Autodesk Fusion 360 part; units mm, degrees
(part 11 of 25)
  arc A1929 (12.5422, 52.0786) -> (12.3177, 51.8541) centre (12.4299, 51.9664) ccw
  arc A1930 (17.6222, 52.0786) -> (17.3977, 51.8541) centre (17.5099, 51.9664) ccw
  line L597 (17.9596, 51.5167) -> (17.51, 51.9663)
  arc A1931 (6.3546, 45.2309) -> (6.0612, 45.3524) centre (6.2079, 45.2917) ccw
  line L598 (10.4521, 47.0845) -> (10.4521, 46.1251)
  arc A1932 (9.1447, 46.0826) -> (9.0232, 45.7892) centre (9.084, 45.9359) ccw
  arc A1933 (18.1777, 51.5103) -> (17.9532, 51.7348) centre (18.0654, 51.6226) ccw
  arc A1934 (5.8229, 44.1544) -> (6.1405, 44.1544) centre (5.9817, 44.1544) ccw
  arc A1935 (9.084, 45.7771) -> (9.084, 46.0946) centre (9.084, 45.9359) ccw
  arc A1936 (17.8473, 51.629) -> (18.0719, 51.4044) centre (17.9596, 51.5167) ccw
  arc A1937 (9.7212, 45.6186) -> (9.9457, 45.3941) centre (9.8334, 45.5063) ccw
  arc A1938 (17.8473, 51.4044) -> (18.0719, 51.629) centre (17.9596, 51.5167) ccw
  arc A1939 (9.0232, 40.5708) -> (9.1447, 40.2774) centre (9.084, 40.4241) ccw
  arc A1940 (6.1405, 42.2056) -> (5.8229, 42.2056) centre (5.9817, 42.2056) ccw
  arc A1941 (9.7212, 45.3941) -> (9.9457, 45.6186) centre (9.8334, 45.5063) ccw
  line L599 (10.4521, 46.1251) -> (9.8334, 45.5064)
  line L600 (13.6189, 52.2351) -> (12.97, 51.9663)
  line L601 (7.172, 40.4241) -> (9.084, 40.4241)
  line L602 (6.6259, 45.7097) -> (6.2079, 45.2917)
  line L603 (5.9817, 44.7456) -> (5.9817, 44.1544)
  arc A1942 (6.5901, 43.0333) -> (6.7116, 43.3267) centre (6.6508, 43.18) ccw
  line L604 (6.6259, 43.1903) -> (6.6508, 43.18)
  arc A1943 (6.0957, 45.4039) -> (6.3202, 45.1794) centre (6.208, 45.2917) ccw
  line L605 (9.6301, 45.7097) -> (9.084, 45.9359)
  arc A1944 (10.3693, 52.113) -> (10.4908, 51.8197) centre (10.4301, 51.9664) ccw
  line L606 (15.51, 51.9663) -> (15.24, 51.6963)
  arc A1945 (6.5652, 45.8563) -> (6.6867, 45.563) centre (6.626, 45.7097) ccw
  line L607 (7.172, 45.9359) -> (6.6259, 45.7097)
  arc A1946 (6.3202, 41.1806) -> (6.0957, 40.956) centre (6.208, 41.0683) ccw
  line L608 (9.084, 45.9359) -> (7.172, 45.9359)
  arc A1947 (6.7116, 43.0333) -> (6.5901, 43.3267) centre (6.6508, 43.18) ccw
  arc A1948 (12.5877, 51.8086) -> (12.8123, 51.5841) centre (12.7, 51.6963) ccw
  line L609 (16.1589, 52.2351) -> (15.51, 51.9663)
  arc A1949 (6.5136, 43.0781) -> (6.7382, 43.3026) centre (6.6259, 43.1904) ccw
  line L610 (9.8334, 45.5064) -> (9.6301, 45.7097)
  line L611 (6.2079, 45.2917) -> (5.9817, 44.7456)
  arc A1950 (9.5693, 45.563) -> (9.6908, 45.8563) centre (9.6301, 45.7097) ccw
  arc A1951 (5.835, 44.8063) -> (6.1284, 44.6848) centre (5.9817, 44.7456) ccw
  arc A1952 (6.1284, 44.2152) -> (5.835, 44.0937) centre (5.9817, 44.1544) ccw
  arc A1953 (14.3819, 52.3818) -> (14.2604, 52.0884) centre (14.3211, 52.2351) ccw
  arc A1954 (15.0822, 52.0786) -> (14.8577, 51.8541) centre (14.9699, 51.9664) ccw
  arc A1955 (15.1277, 51.8086) -> (15.3523, 51.5841) centre (15.24, 51.6963) ccw
  line L612 (11.0789, 52.2351) -> (10.43, 51.9663)
  arc A1956 (7.2328, 45.7892) -> (7.1113, 46.0826) centre (7.1721, 45.9359) ccw
  arc A1957 (6.0612, 43.5476) -> (6.3546, 43.6691) centre (6.2079, 43.6084) ccw
  line L613 (6.6259, 43.1697) -> (6.2079, 42.7517)
  line L614 (6.6508, 43.18) -> (6.6259, 43.1697)
  arc A1958 (9.6908, 40.5036) -> (9.5693, 40.797) centre (9.6301, 40.6503) ccw
  arc A1959 (11.0789, 52.3938) -> (11.0789, 52.0763) centre (11.0789, 52.2351) ccw
  line L615 (9.084, 40.4241) -> (9.6301, 40.6503)
  arc A1960 (6.3202, 43.7206) -> (6.0957, 43.496) centre (6.2079, 43.6083) ccw
  line L616 (5.9817, 44.1544) -> (6.2079, 43.6083)
  arc A1961 (9.084, 40.2654) -> (9.084, 40.5829) centre (9.084, 40.4241) ccw
  line L617 (5.9817, 42.2056) -> (5.9817, 41.6144)
  arc A1962 (6.6867, 40.797) -> (6.5652, 40.5036) centre (6.626, 40.6503) ccw
  line L618 (14.3211, 52.2351) -> (13.6189, 52.2351)
  arc A1963 (7.172, 40.5829) -> (7.172, 40.2654) centre (7.172, 40.4241) ccw
  arc A1964 (10.4908, 47.2403) -> (10.3693, 46.947) centre (10.43, 47.0936) ccw
  line L619 (12.97, 51.9663) -> (12.7, 51.6963)
  arc A1965 (12.9093, 52.113) -> (13.0308, 51.8197) centre (12.9701, 51.9664) ccw
  line L620 (12.43, 51.9663) -> (11.7811, 52.2351)
  arc A1966 (14.9092, 51.8197) -> (15.0307, 52.113) centre (14.97, 51.9663) ccw
  arc A1967 (12.5877, 51.5841) -> (12.8123, 51.8086) centre (12.7, 51.6964) ccw
  arc A1968 (10.5644, 46.0128) -> (10.3398, 46.2373) centre (10.4521, 46.1251) ccw
  arc A1969 (7.172, 46.0946) -> (7.172, 45.7771) centre (7.172, 45.9359) ccw
  line L621 (11.7811, 52.2351) -> (11.0789, 52.2351)
  arc A1970 (14.2402, 42.552) -> (14.3617, 42.2586) centre (14.3009, 42.4053) ccw
  line L622 (6.6259, 35.5497) -> (6.3441, 35.2679)
  arc A1971 (15.746, 44.0556) -> (15.5214, 43.8311) centre (15.6337, 43.9434) ccw
  line L623 (10.7139, 41.081) -> (12.6596, 43.0266)
  arc A1972 (9.9358, 35.0194) -> (10.1603, 35.2439) centre (10.0481, 35.1317) ccw
  arc A1973 (7.1113, 40.2774) -> (7.2328, 40.5708) centre (7.1721, 40.4241) ccw
  arc A1974 (6.5652, 43.3164) -> (6.6866, 43.023) centre (6.6259, 43.1697) ccw
  arc A1975 (6.7382, 45.5974) -> (6.5136, 45.8219) centre (6.6259, 45.7097) ccw
  arc A1976 (9.7423, 45.8219) -> (9.5178, 45.5974) centre (9.63, 45.7097) ccw
  arc A1977 (10.6108, 47.0845) -> (10.2934, 47.0845) centre (10.4521, 47.0845) ccw
  arc A1978 (9.1447, 35.9226) -> (9.0232, 35.6292) centre (9.084, 35.7759) ccw
  arc A1979 (14.8002, 42.7708) -> (15.0247, 42.5463) centre (14.9124, 42.6586) ccw
  arc A1980 (5.835, 42.2663) -> (6.1284, 42.1448) centre (5.9817, 42.2056) ccw
  line L624 (13.4861, 31.4579) -> (10.2148, 34.7291)
  arc A1981 (6.6867, 43.337) -> (6.5651, 43.0437) centre (6.6259, 43.1904) ccw
  line L625 (13.6391, 42.4053) -> (14.3009, 42.4053)
  arc A1982 (9.5693, 35.403) -> (9.6908, 35.6963) centre (9.6301, 35.5496) ccw
  arc A1983 (15.8984, 32.2968) -> (15.6738, 32.5213) centre (15.7861, 32.409) ccw
  line L626 (6.2079, 43.6083) -> (6.6259, 43.1903)
  arc A1984 (14.8349, 31.2991) -> (14.8349, 31.6166) centre (14.8349, 31.4579) ccw
  arc A1985 (6.3546, 42.6909) -> (6.0612, 42.8124) centre (6.2079, 42.7516) ccw
  arc A1986 (9.9119, 41.0909) -> (9.9119, 40.7734) centre (9.9119, 40.9322) ccw
  arc A1987 (6.1405, 44.7456) -> (5.8229, 44.7456) centre (5.9817, 44.7456) ccw
  arc A1988 (6.1284, 41.6752) -> (5.835, 41.5537) centre (5.9817, 41.6144) ccw
  line L627 (9.6301, 35.5497) -> (9.084, 35.7759)
  line L628 (13.0276, 42.6586) -> (13.6391, 42.4053)
  line L629 (5.9817, 41.6144) -> (6.2079, 41.0683)
  line L630 (15.6337, 43.7381) -> (15.6337, 43.9433)
  line L631 (15.7861, 32.4091) -> (14.8349, 31.4579)
  line L632 (9.6301, 40.6503) -> (9.9119, 40.9321)
  line L633 (10.2148, 34.7291) -> (10.0481, 35.1317)
  arc A1989 (6.0957, 42.8639) -> (6.3202, 42.6394) centre (6.208, 42.7517) ccw
  arc A1990 (10.1947, 35.1924) -> (9.9014, 35.0709) centre (10.0481, 35.1317) ccw
  line L634 (9.084, 35.7759) -> (7.172, 35.7759)
  line L635 (6.6259, 40.6503) -> (7.172, 40.4241)
  arc A1991 (7.172, 35.9346) -> (7.172, 35.6171) centre (7.172, 35.7759) ccw
  line L636 (15.3804, 43.1266) -> (15.6337, 43.7381)
  arc A1992 (6.5652, 35.6963) -> (6.6867, 35.403) centre (6.626, 35.5496) ccw
  arc A1993 (6.0612, 41.0076) -> (6.3546, 41.1291) centre (6.2079, 41.0684) ccw
  arc A1994 (10.2934, 46.1251) -> (10.6108, 46.1251) centre (10.4521, 46.1251) ccw
  arc A1995 (10.6017, 41.1932) -> (10.8262, 40.9687) centre (10.714, 41.081) ccw
  arc A1996 (13.6391, 42.5641) -> (13.6391, 42.2466) centre (13.6391, 42.4054) ccw
  arc A1997 (6.5136, 40.5381) -> (6.7382, 40.7626) centre (6.6259, 40.6504) ccw
  line L637 (6.2079, 41.0683) -> (6.6259, 40.6503)
  arc A1998 (6.7382, 43.0574) -> (6.5136, 43.2819) centre (6.6259, 43.1696) ccw
  arc A1999 (10.3545, 40.7734) -> (10.3545, 41.0909) centre (10.3545, 40.9322) ccw
  arc A2000 (14.7227, 31.5702) -> (14.9472, 31.3456) centre (14.8349, 31.4579) ccw
  arc A2001 (13.4861, 31.6166) -> (13.4861, 31.2991) centre (13.4861, 31.4579) ccw
  arc A2002 (12.7718, 42.9144) -> (12.5473, 43.1389) centre (12.6596, 43.0267) ccw
  arc A2003 (15.4927, 43.0143) -> (15.2682, 43.2388) centre (15.3804, 43.1265) ccw
  arc A2004 (5.8229, 41.6144) -> (6.1405, 41.6144) centre (5.9817, 41.6144) ccw
  line L638 (7.172, 35.7759) -> (6.6259, 35.5497)
  arc A2005 (14.9732, 42.5119) -> (14.8517, 42.8052) centre (14.9125, 42.6586) ccw
  line L639 (6.2079, 42.7517) -> (5.9817, 42.2056)
  arc A2006 (9.084, 35.6171) -> (9.084, 35.9346) centre (9.084, 35.7759) ccw
  arc A2007 (7.2328, 35.6292) -> (7.1113, 35.9226) centre (7.172, 35.7759) ccw
  arc A2008 (13.0883, 42.8052) -> (12.9668, 42.5119) centre (13.0276, 42.6586) ccw
  arc A2009 (15.6738, 43.6787) -> (15.8984, 43.9032) centre (15.7861, 43.7909) ccw
  arc A2010 (15.7924, 43.9433) -> (15.4749, 43.9433) centre (15.6337, 43.9433) ccw
  arc A2011 (10.2938, 41.0788) -> (10.4153, 40.7854) centre (10.3546, 40.9321) ccw
  line L640 (21.8221, 44.4397) -> (21.276, 44.6659)
  line L641 (9.9119, 40.9321) -> (10.3545, 40.9321)
  arc A2012 (9.7423, 35.6619) -> (9.5178, 35.4374) centre (9.6301, 35.5496) ccw
  arc A2013 (22.3867, 44.0824) -> (22.0934, 43.9609) centre (22.2401, 44.0217) ccw
  line L642 (10.0481, 35.1317) -> (9.6301, 35.5497)
  line L643 (15.6337, 43.9433) -> (15.7861, 43.7909)
  arc A2014 (10.0682, 34.6684) -> (10.3615, 34.7899) centre (10.2149, 34.7292) ccw
  line L644 (14.8349, 31.4579) -> (13.4861, 31.4579)
  line L645 (10.3545, 40.9321) -> (10.7139, 41.081)
  arc A2015 (15.4749, 43.7381) -> (15.7924, 43.7381) centre (15.6337, 43.7381) ccw
  line L646 (14.9124, 42.6586) -> (15.3804, 43.1266)
  arc A2016 (14.3009, 42.2466) -> (14.3009, 42.5641) centre (14.3009, 42.4054) ccw
  arc A2017 (21.7613, 44.293) -> (21.8828, 44.5863) centre (21.8221, 44.4397) ccw
  arc A2018 (28.3146, 42.5255) -> (27.9971, 42.5255) centre (28.1559, 42.5255) ccw
  arc A2019 (25.3429, 42.5255) -> (25.0253, 42.5255) centre (25.1841, 42.5255) ccw
  line L647 (12.6596, 43.0266) -> (13.0276, 42.6586)
  arc A2020 (21.7364, 42.0567) -> (21.8579, 41.7633) centre (21.7972, 41.91) ccw
  line L648 (21.276, 44.6659) -> (19.364, 44.6659)
  arc A2021 (25.0718, 42.6377) -> (25.2964, 42.4132) centre (25.1841, 42.5255) ccw
  arc A2022 (10.3271, 34.8414) -> (10.1026, 34.6169) centre (10.2149, 34.7292) ccw
  line L649 (22.1039, 41.6179) -> (21.8221, 41.8997)
  arc A2023 (22.3196, 43.4148) -> (22.613, 43.5363) centre (22.4663, 43.4755) ccw
  line L650 (14.3009, 42.4053) -> (14.9124, 42.6586)
  arc A2024 (21.276, 44.5071) -> (21.276, 44.8246) centre (21.276, 44.6658) ccw
  arc A2025 (15.6274, 32.4091) -> (15.9449, 32.4091) centre (15.7862, 32.4091) ccw
  line L651 (15.7861, 43.7909) -> (15.7861, 32.4091)
  arc A2026 (13.3738, 31.3456) -> (13.5983, 31.5702) centre (13.4861, 31.4579) ccw
  arc A2027 (9.5178, 40.7626) -> (9.7423, 40.5381) centre (9.63, 40.6504) ccw
  arc A2028 (25.0253, 41.8071) -> (25.3429, 41.8071) centre (25.1841, 41.8071) ccw
  arc A2029 (21.7098, 42.0326) -> (21.9343, 41.8081) centre (21.8221, 41.9204) ccw
  line L652 (4.8319, 35.2679) -> (4.5501, 35.5497)
  arc A2030 (12.7718, 43.1389) -> (12.5473, 42.9144) centre (12.6595, 43.0267) ccw
  arc A2031 (21.9343, 42.0119) -> (21.7098, 41.7874) centre (21.8221, 41.8997) ccw
  arc A2032 (10.7747, 40.9343) -> (10.6532, 41.2276) centre (10.7139, 41.081) ccw
  line L653 (22.4663, 42.8844) -> (22.4663, 43.4756)
  arc A2033 (10.0241, 40.8198) -> (9.7996, 41.0444) centre (9.9119, 40.9321) ccw
  line L654 (25.1841, 41.8071) -> (24.9949, 41.6179)
  arc A2034 (15.9449, 43.7909) -> (15.6274, 43.7909) centre (15.7862, 43.7909) ccw
  arc A2035 (6.7382, 35.4374) -> (6.5136, 35.6619) centre (6.6259, 35.5496) ccw
  arc A2036 (4.4893, 35.403) -> (4.6108, 35.6963) centre (4.5501, 35.5496) ccw
  arc A2037 (21.9916, 41.5056) -> (22.2161, 41.7301) centre (22.1038, 41.6179) ccw
  arc A2038 (21.9343, 44.5519) -> (21.7098, 44.3274) centre (21.822, 44.4397) ccw
  line L655 (22.2401, 44.0217) -> (21.8221, 44.4397)
  arc A2039 (19.364, 44.8246) -> (19.364, 44.5071) centre (19.364, 44.6658) ccw
  arc A2040 (13.5783, 42.2586) -> (13.6998, 42.552) centre (13.639, 42.4053) ccw
  arc A2041 (12.9153, 42.5463) -> (13.1398, 42.7708) centre (13.0275, 42.6586) ccw
  arc A2042 (15.7804, 43.6773) -> (15.487, 43.7988) centre (15.6337, 43.7381) ccw
  arc A2043 (4.6623, 35.6619) -> (4.4378, 35.4374) centre (4.55, 35.5497) ccw
  arc A2044 (6.2319, 35.3802) -> (6.4564, 35.1556) centre (6.3441, 35.2679) ccw
  line L656 (4.5501, 35.5497) -> (4.004, 35.7759)
  arc A2045 (15.2337, 43.1873) -> (15.5271, 43.0658) centre (15.3804, 43.1266) ccw
  arc A2046 (21.3367, 44.8126) -> (21.2152, 44.5192) centre (21.2759, 44.6659) ccw
  arc A2047 (4.7196, 35.1556) -> (4.9441, 35.3802) centre (4.8319, 35.2679) ccw
  arc A2048 (22.613, 42.8237) -> (22.3196, 42.9452) centre (22.4663, 42.8845) ccw
  arc A2049 (18.9302, 44.3274) -> (18.7056, 44.5519) centre (18.8179, 44.4396) ccw
  arc A2050 (18.7572, 44.5863) -> (18.8787, 44.293) centre (18.8179, 44.4397) ccw
  line L657 (28.1559, 42.5255) -> (27.2855, 43.3959)
  line L658 (25.1841, 42.5255) -> (25.1841, 41.8071)
  arc A2051 (21.8828, 41.7736) -> (21.7614, 42.067) centre (21.8221, 41.9203) ccw
  line L659 (27.2855, 43.3959) -> (26.0545, 43.3959)
  line L660 (6.3441, 35.2679) -> (4.8319, 35.2679)
  line L661 (21.8221, 41.8997) -> (21.7972, 41.91)
  arc A2052 (21.7613, 41.753) -> (21.8828, 42.0463) centre (21.8221, 41.8997) ccw
  arc A2053 (22.1039, 41.7766) -> (22.1039, 41.4591) centre (22.1039, 41.6179) ccw
  arc A2054 (22.3523, 42.226) -> (22.1278, 42.4506) centre (22.24, 42.3383) ccw
  line L662 (24.9949, 41.6179) -> (22.1039, 41.6179)
  arc A2055 (22.0934, 42.3991) -> (22.3867, 42.2776) centre (22.2401, 42.3383) ccw
  arc A2056 (28.0436, 42.4132) -> (28.2682, 42.6377) centre (28.1559, 42.5255) ccw
  arc A2057 (22.3075, 42.8844) -> (22.625, 42.8844) centre (22.4663, 42.8844) ccw
  arc A2058 (4.0647, 35.9226) -> (3.9432, 35.6292) centre (4.004, 35.7759) ccw
  arc A2059 (6.3441, 35.1091) -> (6.3441, 35.4266) centre (6.3441, 35.2678) ccw
  arc A2060 (18.5466, 41.4209) -> (18.2532, 41.5424) centre (18.3999, 41.4817) ccw
  arc A2061 (18.3325, 43.4756) -> (18.0149, 43.4756) centre (18.1737, 43.4756) ccw
  arc A2062 (27.9971, 41.2945) -> (28.3146, 41.2945) centre (28.1559, 41.2945) ccw
  arc A2063 (24.9949, 41.4591) -> (24.9949, 41.7766) centre (24.9949, 41.6179) ccw
  arc A2064 (4.8319, 35.4266) -> (4.8319, 35.1091) centre (4.8319, 35.2678) ccw
  arc A2065 (18.3765, 38.645) -> (18.6594, 38.5008) centre (18.5179, 38.5729) ccw
  line L663 (18.8179, 41.8997) -> (18.3999, 41.4817)
  arc A2066 (18.7474, 38.6736) -> (18.4645, 38.8177) centre (18.606, 38.7457) ccw
  line L664 (18.458, 38.3885) -> (18.4277, 38.197)
  line L665 (21.7972, 41.91) -> (21.8221, 41.9203)
  arc A2067 (22.1278, 43.9094) -> (22.3523, 44.1339) centre (22.2401, 44.0217) ccw
  arc A2068 (27.2855, 43.2371) -> (27.2855, 43.5546) centre (27.2855, 43.3959) ccw
  arc A2069 (18.5865, 38.197) -> (18.269, 38.197) centre (18.4277, 38.197) ccw
  arc A2070 (27.3977, 43.5082) -> (27.1732, 43.2836) centre (27.2855, 43.3959) ccw
  arc A2071 (18.5122, 42.4506) -> (18.2877, 42.226) centre (18.4, 42.3383) ccw
  line L666 (18.4277, 38.197) -> (18.4277, 38.1)
  line L667 (21.8221, 41.9203) -> (22.2401, 42.3383)
  arc A2072 (19.1107, 39.0872) -> (19.2322, 39.3805) centre (19.1715, 39.2339) ccw
  line L668 (26.0545, 43.3959) -> (25.1841, 42.5255)
  arc A2073 (18.3204, 42.9452) -> (18.027, 42.8237) centre (18.1737, 42.8845) ccw
  arc A2074 (24.8827, 41.7302) -> (25.1072, 41.5056) centre (24.9949, 41.6179) ccw
  line L669 (18.8571, 39.0396) -> (18.72, 38.9025)
  arc A2075 (18.8786, 42.067) -> (18.7572, 41.7736) centre (18.8179, 41.9203) ccw
  line L670 (28.1559, 41.2945) -> (28.1559, 42.5255)
  line L671 (19.364, 44.6659) -> (18.8179, 44.4397)
  arc A2076 (26.0545, 43.5546) -> (26.0545, 43.2371) centre (26.0545, 43.3959) ccw
  line L672 (22.2401, 42.3383) -> (22.4663, 42.8844)
  arc A2077 (22.625, 43.4756) -> (22.3075, 43.4756) centre (22.4663, 43.4756) ccw
  arc A2078 (26.1668, 43.2836) -> (25.9423, 43.5082) centre (26.0545, 43.3959) ccw
  arc A2079 (18.2877, 44.1339) -> (18.5122, 43.9094) centre (18.4, 44.0217) ccw
  line L673 (18.518, 38.5729) -> (18.458, 38.3885)
  line L674 (18.1737, 40.9356) -> (18.1737, 40.3444)
  arc A2080 (21.8579, 42.0567) -> (21.7364, 41.7633) centre (21.7972, 41.91) ccw
  arc A2081 (18.269, 38.1) -> (18.5865, 38.1) centre (18.4277, 38.1) ccw
  line L675 (22.4663, 43.4756) -> (22.2401, 44.0217)
  arc A2082 (25.2964, 41.6948) -> (25.0718, 41.9193) centre (25.1841, 41.807) ccw
  arc A2083 (18.027, 43.5363) -> (18.3204, 43.4148) centre (18.1737, 43.4755) ccw
  arc A2084 (18.027, 40.9963) -> (18.3204, 40.8748) centre (18.1737, 40.9356) ccw
  arc A2085 (18.4776, 38.839) -> (18.7344, 38.6523) centre (18.606, 38.7456) ccw
  arc A2086 (18.3071, 38.4375) -> (18.609, 38.3394) centre (18.4581, 38.3885) ccw
  arc A2087 (18.2532, 42.2776) -> (18.5466, 42.3991) centre (18.3999, 42.3383) ccw
  line L676 (21.4533, 36.9584) -> (21.6261, 37.0464)
  arc A2088 (18.2709, 38.2218) -> (18.5845, 38.1721) centre (18.4277, 38.197) ccw
  arc A2089 (19.4248, 44.5192) -> (19.3033, 44.8126) centre (19.364, 44.6659) ccw
  line L677 (19.0139, 39.1536) -> (18.8571, 39.0396)
  arc A2090 (18.6689, 38.5238) -> (18.367, 38.6219) centre (18.518, 38.5729) ccw
  arc A2091 (18.7821, 41.7633) -> (18.9035, 42.0567) centre (18.8428, 41.91) ccw
  arc A2092 (18.3204, 40.4052) -> (18.027, 40.2837) centre (18.1737, 40.3444) ccw
  arc A2093 (19.2435, 39.0924) -> (19.0994, 39.3753) centre (19.1715, 39.2339) ccw
  arc A2094 (18.9302, 41.7874) -> (18.7056, 42.0119) centre (18.8179, 41.8997) ccw
  line L678 (18.606, 38.7457) -> (18.518, 38.5729)
  line L679 (18.8179, 39.3803) -> (19.1715, 39.2339)
  arc A2095 (18.7638, 39.1681) -> (18.9504, 38.9112) centre (18.8571, 39.0397) ccw
  arc A2096 (18.9036, 41.7633) -> (18.7821, 42.0567) centre (18.8429, 41.91) ccw
  line L680 (19.1715, 39.2339) -> (19.0139, 39.1536)
  arc A2097 (18.3325, 40.9356) -> (18.0149, 40.9356) centre (18.1737, 40.9356) ccw
  arc A2098 (18.5466, 43.9609) -> (18.2532, 44.0824) centre (18.3999, 44.0217) ccw
  line L681 (18.3999, 42.3383) -> (18.8179, 41.9203)
  line L682 (18.1737, 40.3444) -> (18.3999, 39.7983)
  arc A2099 (18.7056, 41.8081) -> (18.9302, 42.0326) centre (18.8179, 41.9203) ccw
  arc A2100 (18.0149, 40.3444) -> (18.3325, 40.3444) centre (18.1737, 40.3444) ccw
  line L683 (18.3999, 44.0217) -> (18.1737, 43.4756)
  line L684 (18.3999, 39.7983) -> (18.8179, 39.3803)
  arc A2101 (18.9419, 39.2951) -> (19.086, 39.0122) centre (19.014, 39.1537) ccw
  arc A2102 (19.1073, 39.0252) -> (18.9206, 39.282) centre (19.014, 39.1536) ccw
  arc A2103 (18.8484, 38.8092) -> (18.5915, 38.9958) centre (18.72, 38.9025) ccw
  line L685 (18.1737, 43.4756) -> (18.1737, 42.8844)
  arc A2104 (18.7056, 39.2681) -> (18.9302, 39.4926) centre (18.8179, 39.3803) ccw
  arc A2105 (18.2532, 39.7376) -> (18.5466, 39.8591) centre (18.3999, 39.7984) ccw
  line L686 (18.8179, 41.9203) -> (18.8428, 41.91)
  line L687 (18.72, 38.9025) -> (18.606, 38.7457)
  line L688 (18.3999, 41.4817) -> (18.1737, 40.9356)
  line L689 (18.8428, 41.91) -> (18.8179, 41.8997)
  line L690 (18.8179, 44.4397) -> (18.3999, 44.0217)
  arc A2106 (21.2937, 36.7416) -> (21.244, 37.0552) centre (21.2689, 36.8984) ccw
  arc A2107 (18.7572, 42.0463) -> (18.8787, 41.753) centre (18.818, 41.8997) ccw
  arc A2108 (18.8787, 39.527) -> (18.7572, 39.2336) centre (18.8179, 39.3803) ccw
  arc A2109 (18.9693, 38.9274) -> (18.7448, 39.1519) centre (18.8571, 39.0397) ccw
  arc A2110 (18.0149, 42.8844) -> (18.3325, 42.8844) centre (18.1737, 42.8844) ccw
  arc A2111 (18.5122, 39.9106) -> (18.2877, 39.686) centre (18.4, 39.7983) ccw
  arc A2112 (18.6077, 39.0148) -> (18.8322, 38.7903) centre (18.72, 38.9026) ccw
  arc A2113 (18.6148, 38.3636) -> (18.3012, 38.4133) centre (18.458, 38.3884) ccw
  line L691 (18.1737, 42.8844) -> (18.3999, 42.3383)
  arc A2114 (18.2877, 41.5939) -> (18.5122, 41.3694) centre (18.4, 41.4817) ccw
  arc A2115 (33.9077, 4.9657) -> (34.1322, 4.7412) centre (34.02, 4.8535) ccw
  arc A2116 (21.1166, 13.6842) -> (21.1166, 14.0017) centre (21.1166, 13.843) ccw
  arc A2117 (13.9383, 12.0328) -> (13.6208, 12.0328) centre (13.7796, 12.0328) ccw
  line L692 (33.3711, 4.5847) -> (34.02, 4.8535)
  arc A2118 (13.8918, 10.9141) -> (13.6672, 10.6896) centre (13.7795, 10.8018) ccw
  arc A2119 (34.4478, 4.7412) -> (34.6723, 4.9657) centre (34.5601, 4.8535) ccw
  arc A2120 (35.2089, 4.7435) -> (35.2089, 4.426) centre (35.2089, 4.5848) ccw
  arc A2121 (16.3207, 14.0017) -> (16.3207, 13.6842) centre (16.3207, 13.843) ccw
  line L693 (31.6665, 5.207) -> (32.02, 4.8535)
  arc A2122 (17.1338, 11.4447) -> (16.9093, 11.6693) centre (17.0216, 11.557) ccw
  line L694 (22.559, 12.0525) -> (22.86, 12.3536)
  line L695 (16.3207, 13.843) -> (15.9006, 13.669)
  arc A2123 (16.639, 11.399) -> (16.8636, 11.1745) centre (16.7513, 11.2867) ccw
  line L696 (15.8809, 9.9314) -> (16.7513, 10.8018)
  arc A2124 (21.8174, 11.3983) -> (21.8174, 11.7157) centre (21.8174, 11.557) ccw
  arc A2125 (15.7686, 10.0437) -> (15.9931, 9.8191) centre (15.8808, 9.9314) ccw
  line L697 (34.29, 5.1235) -> (34.56, 4.8535)
  arc A2126 (22.9723, 12.4658) -> (22.7477, 12.2413) centre (22.86, 12.3536) ccw
  arc A2127 (16.8636, 10.6896) -> (16.639, 10.9141) centre (16.7513, 10.8019) ccw
  arc A2128 (22.2982, 11.5843) -> (22.1767, 11.8777) centre (22.2375, 11.731) ccw
  line L698 (13.7795, 10.8018) -> (14.6499, 9.9314)
  arc A2129 (35.1481, 4.438) -> (35.2696, 4.7314) centre (35.2088, 4.5847) ccw
  line L699 (16.7513, 11.2868) -> (17.0215, 11.557)
  arc A2130 (31.6665, 5.0482) -> (31.6665, 5.3658) centre (31.6665, 5.207) ccw
  line L700 (14.6499, 9.9314) -> (15.8809, 9.9314)
  arc A2131 (32.6081, 4.438) -> (32.7296, 4.7314) centre (32.6689, 4.5847) ccw
  line L701 (16.7513, 10.8018) -> (16.7513, 11.2868)
  arc A2132 (15.8809, 9.7727) -> (15.8809, 10.0901) centre (15.8809, 9.9314) ccw
  arc A2133 (21.7566, 11.7037) -> (21.8781, 11.4103) centre (21.8173, 11.557) ccw
  arc A2134 (16.91, 11.2868) -> (16.5925, 11.2868) centre (16.7513, 11.2868) ccw
  line L702 (29.8325, 5.381) -> (30.2526, 5.207)
  line L703 (35.2089, 4.5847) -> (35.9111, 4.5847)
  arc A2135 (29.7203, 5.2688) -> (29.9448, 5.4933) centre (29.8326, 5.3811) ccw
  arc A2136 (34.0807, 4.7068) -> (33.9592, 5.0001) centre (34.02, 4.8535) ccw
  arc A2137 (30.1919, 5.0603) -> (30.3134, 5.3537) centre (30.2527, 5.207) ccw
  line L704 (30.2526, 5.207) -> (31.6665, 5.207)
  arc A2138 (14.5377, 9.8191) -> (14.7622, 10.0437) centre (14.65, 9.9314) ccw
  arc A2139 (16.5925, 10.8018) -> (16.91, 10.8018) centre (16.7513, 10.8018) ccw
  line L705 (21.8174, 11.557) -> (22.2375, 11.731)
  arc A2140 (35.8504, 4.7314) -> (35.9719, 4.438) centre (35.9112, 4.5847) ccw
  arc A2141 (30.2526, 5.3658) -> (30.2526, 5.0482) centre (30.2526, 5.207) ccw
  arc A2142 (22.1252, 11.8433) -> (22.3497, 11.6188) centre (22.2375, 11.731) ccw
  line L706 (32.02, 4.8535) -> (32.6689, 4.5847)
  line L707 (34.56, 4.8535) -> (35.2089, 4.5847)
  arc A2143 (31.9078, 4.7412) -> (32.1323, 4.9657) centre (32.0201, 4.8535) ccw
  arc A2144 (29.8933, 5.5277) -> (29.7718, 5.2343) centre (29.8325, 5.381) ccw
  arc A2145 (36.6207, 4.7068) -> (36.4992, 5.0001) centre (36.56, 4.8534) ccw
  line L708 (22.2375, 11.731) -> (22.559, 12.0525)
  arc A2146 (21.6047, 15.0442) -> (21.8293, 15.2687) centre (21.717, 15.1564) ccw
  arc A2147 (34.4023, 5.0112) -> (34.1777, 5.2357) centre (34.29, 5.1235) ccw
  arc A2148 (32.0808, 5.0001) -> (31.9593, 4.7068) centre (32.0201, 4.8534) ccw
  arc A2149 (31.7787, 5.3193) -> (31.5542, 5.0947) centre (31.6665, 5.207) ccw
  arc A2150 (34.4023, 5.2357) -> (34.1777, 5.0112) centre (34.29, 5.1234) ccw
  line L709 (35.9111, 4.5847) -> (36.56, 4.8535)
  arc A2151 (34.6208, 5.0001) -> (34.4993, 4.7068) centre (34.5601, 4.8535) ccw
  arc A2152 (22.9723, 12.2413) -> (22.7477, 12.4658) centre (22.86, 12.3536) ccw
  line L710 (17.0215, 11.557) -> (21.8174, 11.557)
  arc A2153 (22.4467, 12.1648) -> (22.6712, 11.9403) centre (22.5589, 12.0526) ccw
  arc A2154 (14.6499, 10.0901) -> (14.6499, 9.7727) centre (14.6499, 9.9314) ccw
  line L711 (32.6689, 4.5847) -> (33.3711, 4.5847)
  arc A2155 (35.9111, 4.426) -> (35.9111, 4.7435) centre (35.9111, 4.5848) ccw
  arc A2156 (22.6712, 11.9403) -> (22.4467, 12.1648) centre (22.5589, 12.0526) ccw
  arc A2157 (17.0215, 11.7157) -> (17.0215, 11.3983) centre (17.0215, 11.557) ccw
  line L712 (22.86, 12.3536) -> (29.8325, 5.381)
  arc A2158 (38.1941, 4.9955) -> (38.2438, 4.6819) centre (38.2189, 4.8387) ccw
  line L713 (37.7461, 4.8759) -> (37.9811, 4.8387)
  arc A2159 (38.2588, 6.35) -> (37.9413, 6.35) centre (38.1, 6.35) ccw
  arc A2160 (39.5995, 5.4777) -> (39.375, 5.2532) centre (39.4873, 5.3655) ccw
  arc A2161 (37.5689, 5.1004) -> (37.4708, 4.7984) centre (37.5199, 4.9494) ccw
  arc A2162 (38.6081, 5.0909) -> (38.7522, 4.808) centre (38.6802, 4.9495) ccw
  arc A2163 (37.9412, 4.8387) -> (38.2587, 4.8387) centre (38.0999, 4.8387) ccw
  line L714 (39.4872, 5.3655) -> (39.6555, 5.1972)
  arc A2164 (39.365, 5.2532) -> (39.1405, 5.4777) centre (39.2528, 5.3655) ccw
  line L715 (34.02, 4.8535) -> (34.29, 5.1235)
  arc A2165 (33.3104, 4.7314) -> (33.4319, 4.438) centre (33.3712, 4.5847) ccw
  arc A2166 (38.2189, 4.6799) -> (38.2189, 4.9975) centre (38.2189, 4.8387) ccw
  line L716 (37.1155, 5.1972) -> (37.3079, 5.0574)
  arc A2167 (39.5432, 5.085) -> (39.7677, 5.3095) centre (39.6555, 5.1973) ccw
  arc A2168 (37.9562, 4.6819) -> (38.0059, 4.9955) centre (37.9811, 4.8387) ccw
  arc A2169 (38.1, 6.5087) -> (38.1, 6.1912) centre (38.1, 6.35) ccw
  line L717 (37.9811, 4.8387) -> (38.1, 4.8387)
  arc A2170 (39.9878, 4.808) -> (40.1319, 5.0909) centre (40.0599, 4.9494) ccw
  line L718 (38.1, 4.8387) -> (38.2189, 4.8387)
  line L719 (39.6555, 5.1972) -> (39.8479, 5.0574)
  line L720 (38.1, 4.8387) -> (38.1, 6.35)
  line L721 (37.0096, 5.3031) -> (37.1155, 5.1972)
  line L722 (39.37, 5.5268) -> (39.4872, 5.3655)
  arc A2171 (38.4048, 5.0269) -> (38.503, 4.7249) centre (38.4539, 4.8759) ccw
  arc A2172 (38.9642, 4.916) -> (38.82, 5.1989) centre (38.8921, 5.0575) ccw
  line L723 (38.6801, 4.9494) -> (38.8921, 5.0574)
  line L724 (38.8921, 5.0574) -> (39.0845, 5.1972)
  arc A2173 (39.7488, 5.3257) -> (39.5621, 5.0688) centre (39.6555, 5.1973) ccw
  arc A2174 (37.7709, 5.0327) -> (37.7213, 4.7191) centre (37.7461, 4.8759) ccw
  arc A2175 (37.1219, 5.1908) -> (36.8973, 5.4153) centre (37.0096, 5.3031) ccw
  line L725 (37.3079, 5.0574) -> (37.5199, 4.9494)
  arc A2176 (37.0032, 5.085) -> (37.2277, 5.3095) centre (37.1155, 5.1973) ccw
  line L726 (37.5199, 4.9494) -> (37.7461, 4.8759)
  line L727 (39.8479, 5.0574) -> (40.0599, 4.9494)
  arc A2177 (37.9413, 4.8387) -> (38.2588, 4.8387) centre (38.1, 4.8387) ccw
  arc A2178 (38.7292, 4.7984) -> (38.6311, 5.1004) centre (38.6802, 4.9494) ccw
  arc A2179 (38.1, 4.6799) -> (38.1, 4.9974) centre (38.1, 4.8387) ccw
  arc A2180 (38.9723, 5.3095) -> (39.1968, 5.085) centre (39.0846, 5.1973) ccw
  arc A2181 (38.1, 6.1912) -> (38.1, 6.5087) centre (38.1, 6.35) ccw
  line L728 (40.0599, 4.9494) -> (40.2861, 4.8759)
  arc A2182 (33.3711, 4.426) -> (33.3711, 4.7435) centre (33.3711, 4.5848) ccw
  arc A2183 (38.2587, 6.35) -> (37.9412, 6.35) centre (38.0999, 6.35) ccw
  line L729 (38.4539, 4.8759) -> (38.6801, 4.9494)
  arc A2184 (37.9811, 4.9974) -> (37.9811, 4.68) centre (37.9811, 4.8387) ccw
  arc A2185 (39.7546, 4.929) -> (39.9412, 5.1858) centre (39.8479, 5.0574) ccw
  line L730 (39.2528, 5.3655) -> (39.37, 5.5268)
  arc A2186 (38.4787, 4.7191) -> (38.4291, 5.0327) centre (38.4539, 4.8759) ccw
  arc A2187 (38.7988, 5.1858) -> (38.9854, 4.929) centre (38.8921, 5.0574) ccw
  arc A2188 (39.92, 5.1989) -> (39.7758, 4.916) centre (39.8479, 5.0574) ccw
  arc A2189 (40.237, 4.7249) -> (40.3352, 5.0269) centre (40.2861, 4.8759) ccw
  arc A2190 (39.3588, 5.2721) -> (39.6157, 5.4588) centre (39.4873, 5.3654) ccw
  line L731 (39.0845, 5.1972) -> (39.2528, 5.3655)
  line L732 (36.56, 4.8535) -> (37.0096, 5.3031)
  line L733 (38.1, 6.35) -> (38.1, 4.8387)
  arc A2191 (37.4478, 4.808) -> (37.5919, 5.0909) centre (37.5199, 4.9494) ccw
  arc A2192 (38.1, 4.9975) -> (38.1, 4.6799) centre (38.1, 4.8387) ccw
  arc A2193 (36.4477, 4.9657) -> (36.6722, 4.7412) centre (36.56, 4.8535) ccw
  arc A2194 (39.1243, 5.4588) -> (39.3812, 5.2721) centre (39.2527, 5.3655) ccw
  arc A2195 (32.6689, 4.7435) -> (32.6689, 4.426) centre (32.6689, 4.5848) ccw
  arc A2196 (37.38, 5.1989) -> (37.2358, 4.916) centre (37.3079, 5.0575) ccw
  arc A2197 (37.1219, 5.4153) -> (36.8973, 5.1908) centre (37.0096, 5.303) ccw
  arc A2198 (39.4984, 5.4335) -> (39.2416, 5.6201) centre (39.37, 5.5268) ccw
  arc A2199 (39.4984, 5.6201) -> (39.2416, 5.4335) centre (39.37, 5.5268) ccw
  arc A2200 (37.697, 4.7249) -> (37.7952, 5.0269) centre (37.7461, 4.8759) ccw
  arc A2201 (45.3689, 4.7435) -> (45.3689, 4.426) centre (45.3689, 4.5848) ccw
  line L734 (46.72, 4.8535) -> (46.99, 5.1235)
  line L735 (41.6245, 5.1972) -> (41.7304, 5.3031)
  line L736 (46.99, 5.1235) -> (47.26, 4.8535)
  arc A2202 (46.0711, 4.426) -> (46.0711, 4.7435) centre (46.0711, 4.5848) ccw
  arc A2203 (37.2088, 5.3257) -> (37.0221, 5.0688) centre (37.1155, 5.1973) ccw
  arc A2204 (40.7987, 6.35) -> (40.4812, 6.35) centre (40.6399, 6.35) ccw
  arc A2205 (40.3109, 5.0327) -> (40.2613, 4.7191) centre (40.2861, 4.8759) ccw
  arc A2206 (43.5311, 4.426) -> (43.5311, 4.7435) centre (43.5311, 4.5848) ccw
  arc A2207 (46.0104, 4.7314) -> (46.1319, 4.438) centre (46.0712, 4.5847) ccw
  arc A2208 (41.8426, 5.1908) -> (41.6181, 5.4153) centre (41.7304, 5.3031) ccw
  arc A2209 (40.9448, 5.0269) -> (41.043, 4.7249) centre (40.9939, 4.8759) ccw
  line L737 (43.5311, 4.5847) -> (44.18, 4.8535)
  arc A2210 (40.64, 6.1912) -> (40.64, 6.5087) centre (40.64, 6.35) ccw
  line L738 (44.18, 4.8535) -> (44.45, 5.1235)
  arc A2211 (41.2692, 4.7984) -> (41.1711, 5.1004) centre (41.2202, 4.9494) ccw
  arc A2212 (43.4704, 4.7314) -> (43.5919, 4.438) centre (43.5312, 4.5847) ccw
  arc A2213 (37.2146, 4.929) -> (37.4012, 5.1858) centre (37.3079, 5.0574) ccw
  arc A2214 (41.0187, 4.7191) -> (40.9691, 5.0327) centre (40.9939, 4.8759) ccw
  arc A2215 (40.7589, 4.6799) -> (40.7589, 4.9975) centre (40.7589, 4.8387) ccw
  arc A2216 (41.8426, 5.4153) -> (41.6181, 5.1908) centre (41.7304, 5.303) ccw
  line L739 (40.64, 6.35) -> (40.64, 4.8387)
  arc A2217 (40.64, 6.5087) -> (40.64, 6.1912) centre (40.64, 6.35) ccw
  arc A2218 (40.5211, 4.9974) -> (40.5211, 4.68) centre (40.5211, 4.8387) ccw
  arc A2219 (40.7341, 4.9955) -> (40.7838, 4.6819) centre (40.7589, 4.8387) ccw
  arc A2220 (42.0678, 4.7412) -> (42.2923, 4.9657) centre (42.18, 4.8535) ccw
  arc A2221 (39.1779, 5.0688) -> (38.9912, 5.3257) centre (39.0846, 5.1973) ccw
  arc A2222 (46.6077, 4.9657) -> (46.8322, 4.7412) centre (46.72, 4.8534) ccw
  line L740 (42.18, 4.8535) -> (42.8289, 4.5847)
  line L741 (41.4321, 5.0574) -> (41.6245, 5.1972)
  arc A2223 (44.0677, 4.9657) -> (44.2922, 4.7412) centre (44.18, 4.8535) ccw
  line L742 (44.72, 4.8535) -> (45.3689, 4.5847)
  arc A2224 (41.5042, 4.916) -> (41.36, 5.1989) centre (41.4321, 5.0575) ccw
  arc A2225 (41.7179, 5.0688) -> (41.5312, 5.3257) centre (41.6246, 5.1973) ccw
  arc A2226 (40.64, 4.6799) -> (40.64, 4.9974) centre (40.64, 4.8387) ccw
  line L743 (41.2201, 4.9494) -> (41.4321, 5.0574)
  arc A2227 (42.8289, 4.7435) -> (42.8289, 4.426) centre (42.8289, 4.5848) ccw
  arc A2228 (40.4813, 4.8387) -> (40.7988, 4.8387) centre (40.6401, 4.8387) ccw
  line L744 (44.45, 5.1235) -> (44.72, 4.8535)
  line L745 (38.2189, 4.8387) -> (38.4539, 4.8759)
  line L746 (45.3689, 4.5847) -> (46.0711, 4.5847)
  line L747 (41.7304, 5.3031) -> (42.18, 4.8535)
  arc A2229 (47.1023, 5.0112) -> (46.8777, 5.2357) centre (46.99, 5.1234) ccw
  arc A2230 (44.5623, 5.0112) -> (44.3377, 5.2357) centre (44.45, 5.1234) ccw
  arc A2231 (42.2408, 5.0001) -> (42.1193, 4.7068) centre (42.18, 4.8535) ccw
  arc A2232 (44.2407, 4.7068) -> (44.1192, 5.0001) centre (44.18, 4.8534) ccw
  arc A2233 (41.1481, 5.0909) -> (41.2922, 4.808) centre (41.2202, 4.9494) ccw
  arc A2234 (42.7681, 4.438) -> (42.8896, 4.7314) centre (42.8289, 4.5847) ccw
  line L748 (40.9939, 4.8759) -> (41.2201, 4.9494)
  arc A2235 (40.7988, 6.35) -> (40.4813, 6.35) centre (40.6401, 6.35) ccw
  arc A2236 (46.7807, 4.7068) -> (46.6592, 5.0001) centre (46.7199, 4.8535) ccw
  arc A2237 (41.5123, 5.3095) -> (41.7368, 5.085) centre (41.6246, 5.1973) ccw
  line L749 (42.8289, 4.5847) -> (43.5311, 4.5847)
  arc A2238 (44.6078, 4.7412) -> (44.8323, 4.9657) centre (44.72, 4.8535) ccw
  arc A2239 (40.4962, 4.6819) -> (40.5459, 4.9955) centre (40.5211, 4.8387) ccw
  line L750 (40.2861, 4.8759) -> (40.5211, 4.8387)
  line L751 (46.0711, 4.5847) -> (46.72, 4.8535)
  arc A2240 (44.5623, 5.2357) -> (44.3377, 5.0112) centre (44.45, 5.1234) ccw
  line L752 (40.64, 4.8387) -> (40.7589, 4.8387)
  arc A2241 (40.4812, 4.8387) -> (40.7987, 4.8387) centre (40.6399, 4.8387) ccw
  line L753 (40.64, 4.8387) -> (40.64, 6.35)
  line L754 (40.7589, 4.8387) -> (40.9939, 4.8759)
  line L755 (40.5211, 4.8387) -> (40.64, 4.8387)
  arc A2242 (41.3388, 5.1858) -> (41.5254, 4.929) centre (41.4321, 5.0574) ccw
  line L756 (57.15, 5.1235) -> (57.42, 4.8535)
  arc A2243 (49.3207, 4.7068) -> (49.1992, 5.0001) centre (49.26, 4.8535) ccw
  arc A2244 (51.1511, 4.426) -> (51.1511, 4.7435) centre (51.1511, 4.5848) ccw
  arc A2245 (52.2278, 4.7412) -> (52.4523, 4.9657) centre (52.34, 4.8535) ccw
  line L757 (51.8, 4.8535) -> (52.07, 5.1235)
  line L758 (49.53, 5.1235) -> (49.8, 4.8535)
  arc A2246 (52.4008, 5.0001) -> (52.2793, 4.7068) centre (52.34, 4.8535) ccw
  line L759 (53.6911, 4.5847) -> (54.34, 4.8535)
  arc A2247 (49.1477, 4.9657) -> (49.3722, 4.7412) centre (49.26, 4.8535) ccw
  arc A2248 (51.6877, 4.9657) -> (51.9122, 4.7412) centre (51.7999, 4.8535) ccw
  line L760 (54.88, 4.8535) -> (55.5289, 4.5847)
  line L761 (50.4489, 4.5847) -> (51.1511, 4.5847)
  arc A2249 (40.64, 4.9975) -> (40.64, 4.6799) centre (40.64, 4.8387) ccw
  arc A2250 (45.3081, 4.438) -> (45.4296, 4.7314) centre (45.3688, 4.5847) ccw
  arc A2251 (54.7223, 5.2357) -> (54.4977, 5.0112) centre (54.61, 5.1234) ccw
  arc A2252 (56.9407, 4.7068) -> (56.8192, 5.0001) centre (56.88, 4.8535) ccw
  arc A2253 (58.0081, 4.438) -> (58.1296, 4.7314) centre (58.0689, 4.5847) ccw
  arc A2254 (44.7808, 5.0001) -> (44.6593, 4.7068) centre (44.7201, 4.8535) ccw
  arc A2255 (40.1089, 5.1004) -> (40.0108, 4.7984) centre (40.0599, 4.9494) ccw
  line L762 (52.07, 5.1235) -> (52.34, 4.8535)
  line L763 (52.34, 4.8535) -> (52.9889, 4.5847)
  arc A2256 (49.6878, 4.7412) -> (49.9123, 4.9657) centre (49.8, 4.8535) ccw
  arc A2257 (47.8481, 4.438) -> (47.9696, 4.7314) centre (47.9089, 4.5847) ccw
  arc A2258 (55.4681, 4.438) -> (55.5896, 4.7314) centre (55.5288, 4.5847) ccw
  arc A2259 (47.9089, 4.7435) -> (47.9089, 4.426) centre (47.9089, 4.5848) ccw
  arc A2260 (47.1478, 4.7412) -> (47.3723, 4.9657) centre (47.2601, 4.8534) ccw
  arc A2261 (57.2623, 5.0112) -> (57.0377, 5.2357) centre (57.15, 5.1234) ccw
  arc A2262 (57.3078, 4.7412) -> (57.5323, 4.9657) centre (57.4201, 4.8534) ccw
  arc A2263 (57.2623, 5.2357) -> (57.0377, 5.0112) centre (57.15, 5.1234) ccw
  line L764 (57.42, 4.8535) -> (58.0689, 4.5847)
  arc A2264 (49.6423, 5.0112) -> (49.4177, 5.2357) centre (49.53, 5.1234) ccw
  arc A2265 (49.6423, 5.2357) -> (49.4177, 5.0112) centre (49.53, 5.1234) ccw
  line L765 (52.9889, 4.5847) -> (53.6911, 4.5847)
  arc A2266 (52.9889, 4.7435) -> (52.9889, 4.426) centre (52.9889, 4.5848) ccw
  line L766 (54.34, 4.8535) -> (54.61, 5.1235)
  arc A2267 (53.6911, 4.426) -> (53.6911, 4.7435) centre (53.6911, 4.5848) ccw
  arc A2268 (48.5504, 4.7314) -> (48.6719, 4.438) centre (48.6112, 4.5847) ccw
  arc A2269 (56.1704, 4.7314) -> (56.2919, 4.438) centre (56.2311, 4.5847) ccw
  line L767 (48.6111, 4.5847) -> (49.26, 4.8535)
  arc A2270 (52.1823, 5.0112) -> (51.9577, 5.2357) centre (52.07, 5.1234) ccw
  arc A2271 (56.2311, 4.426) -> (56.2311, 4.7435) centre (56.2311, 4.5848) ccw
  arc A2272 (56.7677, 4.9657) -> (56.9922, 4.7412) centre (56.88, 4.8534) ccw
  line L768 (55.5289, 4.5847) -> (56.2311, 4.5847)
  line L769 (51.1511, 4.5847) -> (51.8, 4.8535)
  arc A2273 (50.4489, 4.7435) -> (50.4489, 4.426) centre (50.4489, 4.5848) ccw
  line L770 (56.88, 4.8535) -> (57.15, 5.1235)
  arc A2274 (53.6304, 4.7314) -> (53.7519, 4.438) centre (53.6912, 4.5847) ccw
  line L771 (49.26, 4.8535) -> (49.53, 5.1235)
  arc A2275 (49.8608, 5.0001) -> (49.7393, 4.7068) centre (49.8, 4.8535) ccw
  arc A2276 (51.8607, 4.7068) -> (51.7392, 5.0001) centre (51.7999, 4.8534) ccw
  arc A2277 (54.7223, 5.0112) -> (54.4977, 5.2357) centre (54.61, 5.1234) ccw
  arc A2278 (47.3208, 5.0001) -> (47.1993, 4.7068) centre (47.2601, 4.8534) ccw
  arc A2279 (54.2277, 4.9657) -> (54.4522, 4.7412) centre (54.3399, 4.8535) ccw
  arc A2280 (55.5289, 4.7435) -> (55.5289, 4.426) centre (55.5289, 4.5848) ccw
  arc A2281 (50.3881, 4.438) -> (50.5096, 4.7314) centre (50.4489, 4.5847) ccw
  arc A2282 (54.9408, 5.0001) -> (54.8193, 4.7068) centre (54.8801, 4.8535) ccw
  line L772 (56.2311, 4.5847) -> (56.88, 4.8535)
  arc A2283 (47.1023, 5.2357) -> (46.8777, 5.0112) centre (46.99, 5.1234) ccw
  line L773 (47.9089, 4.5847) -> (48.6111, 4.5847)
  line L774 (49.8, 4.8535) -> (50.4489, 4.5847)
  arc A2284 (51.0904, 4.7314) -> (51.2119, 4.438) centre (51.1512, 4.5847) ccw
  arc A2285 (54.7678, 4.7412) -> (54.9923, 4.9657) centre (54.8801, 4.8534) ccw
  line L775 (47.26, 4.8535) -> (47.9089, 4.5847)
  line L776 (63.8511, 4.5847) -> (64.5, 4.8535)
  arc A2286 (64.8823, 5.2357) -> (64.6577, 5.0112) centre (64.77, 5.1235) ccw
  arc A2287 (61.3111, 4.426) -> (61.3111, 4.7435) centre (61.3111, 4.5848) ccw
  arc A2288 (48.6111, 4.426) -> (48.6111, 4.7435) centre (48.6111, 4.5848) ccw
  arc A2289 (52.9281, 4.438) -> (53.0496, 4.7314) centre (52.9888, 4.5847) ccw
  line L777 (54.61, 5.1235) -> (54.88, 4.8535)
  arc A2290 (59.8023, 5.0112) -> (59.5777, 5.2357) centre (59.69, 5.1234) ccw
  arc A2291 (68.1681, 4.438) -> (68.2896, 4.7314) centre (68.2288, 4.5847) ccw
  line L778 (65.04, 4.8535) -> (65.6889, 4.5847)
  arc A2292 (67.1007, 4.7068) -> (66.9792, 5.0001) centre (67.04, 4.8535) ccw
  arc A2293 (68.2289, 4.7435) -> (68.2289, 4.426) centre (68.2289, 4.5848) ccw
  arc A2294 (62.3423, 5.0112) -> (62.1177, 5.2357) centre (62.23, 5.1234) ccw
  arc A2295 (63.7904, 4.7314) -> (63.9119, 4.438) centre (63.8512, 4.5847) ccw
  line L779 (59.96, 4.8535) -> (60.6089, 4.5847)
  arc A2296 (62.3878, 4.7412) -> (62.6123, 4.9657) centre (62.5001, 4.8535) ccw
  arc A2297 (67.4223, 5.2357) -> (67.1977, 5.0112) centre (67.31, 5.1234) ccw
  arc A2298 (57.4808, 5.0001) -> (57.3593, 4.7068) centre (57.4201, 4.8534) ccw
  arc A2299 (59.8478, 4.7412) -> (60.0723, 4.9657) centre (59.9601, 4.8535) ccw
  arc A2300 (66.3304, 4.7314) -> (66.4519, 4.438) centre (66.3912, 4.5847) ccw
  arc A2301 (64.5607, 4.7068) -> (64.4392, 5.0001) centre (64.4999, 4.8535) ccw
  arc A2302 (61.8477, 4.9657) -> (62.0722, 4.7412) centre (61.9599, 4.8535) ccw
  line L780 (58.0689, 4.5847) -> (58.7711, 4.5847)
  arc A2303 (63.0881, 4.438) -> (63.2096, 4.7314) centre (63.1489, 4.5847) ccw
  line L781 (64.77, 5.1235) -> (65.04, 4.8535)
  arc A2304 (59.3077, 4.9657) -> (59.5322, 4.7412) centre (59.42, 4.8535) ccw
  arc A2305 (59.8023, 5.2357) -> (59.5777, 5.0112) centre (59.69, 5.1234) ccw
  arc A2306 (60.6089, 4.7435) -> (60.6089, 4.426) centre (60.6089, 4.5848) ccw
  arc A2307 (67.4223, 5.0112) -> (67.1977, 5.2357) centre (67.31, 5.1234) ccw
  arc A2308 (62.3423, 5.2357) -> (62.1177, 5.0112) centre (62.23, 5.1234) ccw
  arc A2309 (66.9277, 4.9657) -> (67.1522, 4.7412) centre (67.04, 4.8535) ccw
  arc A2310 (58.7104, 4.7314) -> (58.8319, 4.438) centre (58.7711, 4.5847) ccw
  line L782 (59.69, 5.1235) -> (59.96, 4.8535)
  arc A2311 (64.3877, 4.9657) -> (64.6122, 4.7412) centre (64.5, 4.8535) ccw
  line L783 (65.6889, 4.5847) -> (66.3911, 4.5847)
  line L784 (59.42, 4.8535) -> (59.69, 5.1235)
  arc A2312 (64.9278, 4.7412) -> (65.1523, 4.9657) centre (65.0401, 4.8535) ccw
  line L785 (67.58, 4.8535) -> (68.2289, 4.5847)
  line L786 (63.1489, 4.5847) -> (63.8511, 4.5847)
  arc A2313 (54.4007, 4.7068) -> (54.2792, 5.0001) centre (54.34, 4.8535) ccw
  line L787 (67.04, 4.8535) -> (67.31, 5.1235)
  arc A2314 (59.4807, 4.7068) -> (59.3592, 5.0001) centre (59.42, 4.8535) ccw
  line L788 (58.7711, 4.5847) -> (59.42, 4.8535)
  arc A2315 (62.0207, 4.7068) -> (61.8992, 5.0001) centre (61.96, 4.8534) ccw
  arc A2316 (58.7711, 4.426) -> (58.7711, 4.7435) centre (58.7711, 4.5848) ccw
  line L789 (66.3911, 4.5847) -> (67.04, 4.8535)
  arc A2317 (62.5608, 5.0001) -> (62.4393, 4.7068) centre (62.5001, 4.8535) ccw
  arc A2318 (65.6281, 4.438) -> (65.7496, 4.7314) centre (65.6889, 4.5847) ccw
  arc A2319 (64.8823, 5.0112) -> (64.6577, 5.2357) centre (64.77, 5.1235) ccw
  line L790 (62.23, 5.1235) -> (62.5, 4.8535)
  arc A2320 (63.8511, 4.426) -> (63.8511, 4.7435) centre (63.8511, 4.5848) ccw
  arc A2321 (65.6889, 4.7435) -> (65.6889, 4.426) centre (65.6889, 4.5848) ccw
  arc A2322 (67.6408, 5.0001) -> (67.5193, 4.7068) centre (67.58, 4.8534) ccw
  line L791 (60.6089, 4.5847) -> (61.3111, 4.5847)
  arc A2323 (61.2504, 4.7314) -> (61.3719, 4.438) centre (61.3112, 4.5847) ccw
  arc A2324 (66.3911, 4.426) -> (66.3911, 4.7435) centre (66.3911, 4.5848) ccw
  arc A2325 (65.1008, 5.0001) -> (64.9793, 4.7068) centre (65.0401, 4.8534) ccw
  arc A2326 (68.9311, 4.426) -> (68.9311, 4.7435) centre (68.9311, 4.5848) ccw
  line L792 (67.31, 5.1235) -> (67.58, 4.8535)
  line L793 (64.5, 4.8535) -> (64.77, 5.1235)
  arc A2327 (52.1823, 5.2357) -> (51.9577, 5.0112) centre (52.07, 5.1234) ccw
  line L794 (68.2289, 4.5847) -> (68.9311, 4.5847)
  arc A2328 (60.0208, 5.0001) -> (59.8993, 4.7068) centre (59.9601, 4.8535) ccw
  arc A2329 (64.6577, 7.6888) -> (64.8823, 7.4643) centre (64.77, 7.5766) ccw
  line L795 (70.3453, 5.9989) -> (70.3453, 6.7011)
  arc A2330 (64.6577, 7.4643) -> (64.8823, 7.6888) centre (64.77, 7.5766) ccw
  line L796 (64.5, 7.8465) -> (63.8511, 8.1153)
  line L797 (69.58, 4.8535) -> (70.0765, 5.35)
  arc A2331 (68.9919, 8.262) -> (68.8704, 7.9686) centre (68.9312, 8.1153) ccw
  line L798 (68.2289, 8.1153) -> (67.58, 7.8465)
  arc A2332 (63.8511, 7.9565) -> (63.8511, 8.274) centre (63.8511, 8.1152) ccw
  arc A2333 (67.1977, 7.6888) -> (67.4223, 7.4643) centre (67.31, 7.5766) ccw
  line L799 (61.96, 4.8535) -> (62.23, 5.1235)
  arc A2334 (67.1522, 7.9588) -> (66.9277, 7.7343) centre (67.04, 7.8465) ccw
  arc A2335 (66.9792, 7.6999) -> (67.1007, 7.9932) centre (67.04, 7.8466) ccw
  line L800 (62.5, 4.8535) -> (63.1489, 4.5847)
  arc A2336 (63.9119, 8.262) -> (63.7904, 7.9686) centre (63.8512, 8.1153) ccw
  arc A2337 (67.6923, 7.7343) -> (67.4678, 7.9588) centre (67.58, 7.8465) ccw
  arc A2338 (62.6123, 7.7343) -> (62.3878, 7.9588) centre (62.5001, 7.8466) ccw
  arc A2339 (67.5193, 7.9932) -> (67.6408, 7.6999) centre (67.58, 7.8466) ccw
  arc A2340 (69.9643, 7.2377) -> (70.1888, 7.4622) centre (70.0765, 7.35) ccw
  arc A2341 (70.1888, 5.2378) -> (69.9643, 5.4623) centre (70.0765, 5.3501) ccw
  arc A2342 (66.4519, 8.262) -> (66.3304, 7.9686) centre (66.3912, 8.1153) ccw
  arc A2343 (62.4393, 7.9932) -> (62.5608, 7.6999) centre (62.5001, 7.8466) ccw
  arc A2344 (69.6922, 7.9588) -> (69.4677, 7.7343) centre (69.5799, 7.8465) ccw
  line L801 (68.9311, 4.5847) -> (69.58, 4.8535)
  arc A2345 (63.1489, 4.7435) -> (63.1489, 4.426) centre (63.1489, 4.5848) ccw
  line L802 (62.23, 7.5765) -> (61.96, 7.8465)
  arc A2346 (62.1177, 7.4643) -> (62.3423, 7.6888) centre (62.23, 7.5765) ccw
  arc A2347 (64.6122, 7.9588) -> (64.3877, 7.7343) centre (64.5, 7.8465) ccw
  line L803 (67.58, 7.8465) -> (67.31, 7.5765)
  arc A2348 (63.2096, 7.9686) -> (63.0881, 8.262) centre (63.1489, 8.1153) ccw
  line L804 (69.58, 7.8465) -> (68.9311, 8.1153)
  arc A2349 (70.2232, 7.4107) -> (69.9299, 7.2892) centre (70.0766, 7.35) ccw
  line L805 (63.8511, 8.1153) -> (63.1489, 8.1153)
  line L806 (62.5, 7.8465) -> (62.23, 7.5765)
  arc A2350 (68.9311, 7.9565) -> (68.9311, 8.274) centre (68.9311, 8.1152) ccw
  arc A2351 (62.0722, 7.9588) -> (61.8477, 7.7343) centre (61.9599, 7.8466) ccw
  arc A2352 (68.8704, 4.7314) -> (68.9919, 4.438) centre (68.9312, 4.5847) ccw
  arc A2353 (69.5192, 7.6999) -> (69.6407, 7.9932) centre (69.5799, 7.8465) ccw
  line L807 (67.04, 7.8465) -> (66.3911, 8.1153)
  line L808 (64.77, 7.5765) -> (64.5, 7.8465)
  line L809 (61.96, 7.8465) -> (61.3111, 8.1153)
  line L810 (70.0765, 5.35) -> (70.3453, 5.9989)
  line L811 (61.3111, 4.5847) -> (61.96, 4.8535)
  arc A2354 (70.492, 5.9381) -> (70.1986, 6.0596) centre (70.3453, 5.9989) ccw
  arc A2355 (60.5481, 4.438) -> (60.6696, 4.7314) centre (60.6089, 4.5847) ccw
  line L812 (63.1489, 8.1153) -> (62.5, 7.8465)
  line L813 (68.9311, 8.1153) -> (68.2289, 8.1153)
  arc A2356 (69.9299, 5.4108) -> (70.2232, 5.2893) centre (70.0766, 5.35) ccw
  arc A2357 (67.4678, 4.7412) -> (67.6923, 4.9657) centre (67.58, 4.8534) ccw
  arc A2358 (58.0689, 4.7435) -> (58.0689, 4.426) centre (58.0689, 4.5848) ccw
  line L814 (65.6889, 8.1153) -> (65.04, 7.8465)
  arc A2359 (65.1523, 7.7343) -> (64.9278, 7.9588) centre (65.0401, 7.8465) ccw
  arc A2360 (64.4392, 7.6999) -> (64.5607, 7.9932) centre (64.4999, 7.8466) ccw
  arc A2361 (70.1986, 6.6404) -> (70.492, 6.7619) centre (70.3453, 6.7012) ccw
  arc A2362 (70.504, 6.7011) -> (70.1865, 6.7011) centre (70.3453, 6.7011) ccw
  line L815 (70.3453, 6.7011) -> (70.0765, 7.35)
  arc A2363 (62.1177, 7.6888) -> (62.3423, 7.4643) centre (62.23, 7.5765) ccw
  arc A2364 (63.1489, 8.274) -> (63.1489, 7.9565) centre (63.1489, 8.1152) ccw
  arc A2365 (69.4677, 4.9657) -> (69.6922, 4.7412) centre (69.5799, 4.8534) ccw
  arc A2366 (68.2896, 7.9686) -> (68.1681, 8.262) centre (68.2288, 8.1153) ccw
  arc A2367 (70.1865, 5.9989) -> (70.504, 5.9989) centre (70.3453, 5.9989) ccw
  arc A2368 (68.2289, 8.274) -> (68.2289, 7.9565) centre (68.2289, 8.1152) ccw
  line L816 (57.15, 7.5765) -> (56.88, 7.8465)
  line L817 (52.34, 7.8465) -> (52.07, 7.5765)
  arc A2369 (64.9793, 7.9932) -> (65.1008, 7.6999) centre (65.0401, 7.8466) ccw
  arc A2370 (66.3911, 7.9565) -> (66.3911, 8.274) centre (66.3911, 8.1152) ccw
  line L818 (59.42, 7.8465) -> (58.7711, 8.1153)
  arc A2371 (52.2793, 7.9932) -> (52.4008, 7.6999) centre (52.34, 7.8465) ccw
  arc A2372 (69.6407, 4.7068) -> (69.5192, 5.0001) centre (69.5799, 4.8535) ccw
  arc A2373 (60.6089, 8.274) -> (60.6089, 7.9565) centre (60.6089, 8.1152) ccw
  arc A2374 (51.9577, 7.6888) -> (52.1823, 7.4643) centre (52.07, 7.5765) ccw
  arc A2375 (58.0689, 8.274) -> (58.0689, 7.9565) centre (58.0689, 8.1152) ccw
  arc A2376 (51.9122, 7.9588) -> (51.6877, 7.7343) centre (51.7999, 7.8466) ccw
  arc A2377 (59.5777, 7.4643) -> (59.8023, 7.6888) centre (59.69, 7.5766) ccw
  line L819 (56.2311, 8.1153) -> (55.5289, 8.1153)
  arc A2378 (53.0496, 7.9686) -> (52.9281, 8.262) centre (52.9888, 8.1153) ccw
  arc A2379 (60.0723, 7.7343) -> (59.8478, 7.9588) centre (59.9601, 7.8465) ccw
  arc A2380 (52.4523, 7.7343) -> (52.2278, 7.9588) centre (52.34, 7.8466) ccw
  line L820 (66.3911, 8.1153) -> (65.6889, 8.1153)
  arc A2381 (52.9889, 8.274) -> (52.9889, 7.9565) centre (52.9889, 8.1152) ccw
  line L821 (60.6089, 8.1153) -> (59.96, 7.8465)
  arc A2382 (58.7711, 7.9565) -> (58.7711, 8.274) centre (58.7711, 8.1152) ccw
  line L822 (67.31, 7.5765) -> (67.04, 7.8465)
  line L823 (51.8, 7.8465) -> (51.1511, 8.1153)
  arc A2383 (57.0377, 7.4643) -> (57.2623, 7.6888) centre (57.15, 7.5766) ccw
  line L824 (65.04, 7.8465) -> (64.77, 7.5765)
  arc A2384 (55.5896, 7.9686) -> (55.4681, 8.262) centre (55.5288, 8.1153) ccw
  line L825 (51.1511, 8.1153) -> (50.4489, 8.1153)
  arc A2385 (56.9922, 7.9588) -> (56.7677, 7.7343) centre (56.88, 7.8465) ccw
  arc A2386 (50.4489, 8.274) -> (50.4489, 7.9565) centre (50.4489, 8.1152) ccw
  line L826 (54.88, 7.8465) -> (54.61, 7.5765)
  arc A2387 (54.8193, 7.9932) -> (54.9408, 7.6999) centre (54.8801, 7.8466) ccw
  arc A2388 (65.7496, 7.9686) -> (65.6281, 8.262) centre (65.6889, 8.1153) ccw
  arc A2389 (59.3592, 7.6999) -> (59.4807, 7.9932) centre (59.42, 7.8466) ccw
  arc A2390 (56.2311, 7.9565) -> (56.2311, 8.274) centre (56.2311, 8.1152) ccw
  line L827 (52.9889, 8.1153) -> (52.34, 7.8465)
  arc A2391 (57.0377, 7.6888) -> (57.2623, 7.4643) centre (57.15, 7.5766) ccw
  arc A2392 (61.8992, 7.6999) -> (62.0207, 7.9932) centre (61.9599, 7.8466) ccw
  arc A2393 (51.2119, 8.262) -> (51.0904, 7.9686) centre (51.1512, 8.1153) ccw
  arc A2394 (56.8192, 7.6999) -> (56.9407, 7.9932) centre (56.88, 7.8465) ccw
  arc A2395 (59.5322, 7.9588) -> (59.3077, 7.7343) centre (59.42, 7.8465) ccw
  arc A2396 (57.3593, 7.9932) -> (57.4808, 7.6999) centre (57.4201, 7.8466) ccw
  arc A2397 (58.8319, 8.262) -> (58.7104, 7.9686) centre (58.7711, 8.1153) ccw
  line L828 (54.61, 7.5765) -> (54.34, 7.8465)
  arc A2398 (59.5777, 7.6888) -> (59.8023, 7.4643) centre (59.69, 7.5766) ccw
  arc A2399 (55.5289, 8.274) -> (55.5289, 7.9565) centre (55.5289, 8.1152) ccw
  line L829 (58.7711, 8.1153) -> (58.0689, 8.1153)
  line L830 (59.96, 7.8465) -> (59.69, 7.5765)
  arc A2400 (67.1977, 7.4643) -> (67.4223, 7.6888) centre (67.31, 7.5766) ccw
  arc A2401 (59.8993, 7.9932) -> (60.0208, 7.6999) centre (59.9601, 7.8466) ccw
  line L831 (70.0765, 7.35) -> (69.58, 7.8465)
  arc A2402 (54.4977, 7.6888) -> (54.7223, 7.4643) centre (54.61, 7.5766) ccw
  arc A2403 (51.9577, 7.4643) -> (52.1823, 7.6888) centre (52.07, 7.5765) ccw
  arc A2404 (51.7392, 7.6999) -> (51.8607, 7.9932) centre (51.7999, 7.8466) ccw
  arc A2405 (56.2919, 8.262) -> (56.1704, 7.9686) centre (56.2311, 8.1153) ccw
  line L832 (55.5289, 8.1153) -> (54.88, 7.8465)